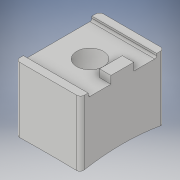
# Autodesk Inventor part: upper_fender_spacer
Saved by Autodesk Inventor 2019 (Build 230136000, 136)
## iProperties
Created: 2019-10-03
Part Number: upper_fender_spacer
Material: Generic
Document SubType Name: Modeling
Designer: Alex
Density: 1 g/cm^3
Appearance: Default
Author: Alex
Autodesk Inventor part; units mm, degrees
ref_plane "YZ Plane" through (0, 0, 0) normal (1, 0, 0) x (0, 1, 0)
ref_plane "XZ Plane" through (0, 0, 0) normal (0, 1, 0) x (-1, 0, 0)
ref_plane "XY Plane" through (0, 0, 0) normal (0, 0, 1) x (1, 0, 0)
sketch "Sketch1" plane through (0, 0, 0) normal (0, 1, 0) x (-1, 0, 0)
  line L0 (5.233, 7.4455) -> (-11.767, 7.4455)
  line L1 (-11.767, 7.4455) -> (-11.767, -14.5545)
  line L2 (-11.767, -14.5545) -> (5.233, -14.5545)
  circle A0 centre (-3.267, -3.5545) radius 3.5
  line L3 (5.233, 7.4455) -> (5.233, -14.5545)
  point P0 (0, 0)
  dimension "d2" = 22
  dimension "d3" = 17
  dimension "d8" = 7
  dimension "d10" = 11
  dimension "d11" = 8.5
  constraints: 8 end point, 1 centre point, 1 horizontal, 1 parallel, 1 perpendicular, 1 vertical
  measures "d2" distance of L2.end L0.start
  measures "d3" distance of L0.start L0.end
  measures "d8" diameter of A0
  measures "d10" distance from line of A0.centre L0
  measures "d11" distance from line of A0.centre L3
extrude "Extrusion1" add sketch "Sketch1" along normal blind 20
sketch "Sketch2" plane through (0, 20, 0) normal (0, 1, 0) x (1, 0, 0)
  line L0 (-5.233, -7.4455) -> (11.767, -7.4455) projected
  line L1 (11.767, -7.4455) -> (11.767, 14.5545) projected
  line L2 (-5.233, -7.4455) -> (11.767, -7.4455)
  line L3 (11.767, -7.4455) -> (11.767, -5.4455)
  line L4 (11.767, -5.4455) -> (-5.233, -5.4455)
  line L5 (-5.233, -5.4455) -> (-5.233, -7.4455)
  line L6 (-5.233, 14.5545) -> (-5.233, -7.4455) projected
  line L7 (-5.233, 14.5545) -> (11.767, 14.5545)
  line L8 (11.767, 14.5545) -> (11.767, 12.5545)
  line L9 (11.767, 12.5545) -> (-5.233, 12.5545)
  line L10 (-5.233, 12.5545) -> (-5.233, 14.5545)
  line L11 (11.767, 0.5545) -> (8.767, 0.5545)
  line L12 (8.767, 0.5545) -> (8.767, 6.5545)
  line L13 (8.767, 6.5545) -> (11.767, 6.5545)
  line L14 (11.767, 6.5545) -> (11.767, 0.5545)
  line L15 (11.767, 0.5545) -> (8.767, 0.5545)
  line L16 (8.767, 0.5545) -> (8.767, 6.5545)
  line L17 (8.767, 6.5545) -> (11.767, 6.5545)
  line L18 (11.767, 6.5545) -> (11.767, 0.5545)
  point P0 (0, 0)
  dimension "d14" = 2
  dimension "d15" = 2
  dimension "d16" = 3
  dimension "d17" = 6
  dimension "d18" = 8
  constraints: 32 end point, 8 parallel, 4 horizontal, 4 perpendicular, 3 point on line
  measures "d14" distance between parallel lines of L4 L0
  measures "d15" distance between parallel lines of L7 L9
  measures "d16" distance between parallel lines of L1 L12
  measures "d17" distance between parallel lines of L11 L13
  measures "d18" distance between parallel lines of L11 L0
extrude "Extrusion2" add sketch "Sketch2" along normal blind 1 contours L5 L4 L1 L0 | L6 L7 L1 L9
sketch "Sketch3" plane through (0, 20, 0) normal (0, 1, 0) x (1, 0, 0)
  line L0 (11.767, -5.4455) -> (11.767, 12.5545) projected
  line L1 (11.767, 0.5545) -> (8.767, 0.5545)
  line L2 (8.767, 0.5545) -> (8.767, 6.5545)
  line L3 (8.767, 6.5545) -> (11.767, 6.5545)
  line L4 (11.767, 6.5545) -> (11.767, 0.5545)
  line L5 (-5.233, -7.4455) -> (11.767, -7.4455) projected
  point P0 (0, 0)
  dimension "d21" = 6
  dimension "d22" = 3
  dimension "d23" = 8
  constraints: 8 end point, 2 parallel, 1 horizontal, 1 perpendicular, 1 point on line
  measures "d21" distance between parallel lines of L3 L1
  measures "d22" distance between parallel lines of L0 L2
  measures "d23" distance between parallel lines of L1 L5
extrude "Extrusion3" add sketch "Sketch3" along normal blind 2
sketch "Sketch5" plane through (-5.233, 0, -14.5545) normal (-1, 0, 0) x (0, 0, 1)
  line L0 (-21.5, -5) -> (43.5, -5)
  line L1 (11, -5) -> (11, 5)
  line L2 (0, 0) -> (0, 21) projected
  arc A0 (43.5, -5) -> (22, 3.9439) centre (11, -52.8125) ccw
  line L3 (2, 20) -> (20, 20) projected
  arc A1 (11, 5) -> (-21.5, -5) centre (11, -52.8125) ccw
  arc A2 (0, 3.9439) -> (-21.5, -5) centre (11, -52.8125) ccw
  line L4 (0, 0) -> (22, 0) projected
  line L5 (22, 0) -> (22, 3.9439)
  line L6 (22, 0) -> (0, 0)
  line L7 (0, 0) -> (0, 3.9439)
  arc A3 (22, 3.9439) -> (11, 5) centre (11, -52.8125) ccw
  line L8 (-15.7774, -378) -> (53.3664, -378)
  point P0 (14.5545, 0)
  dimension "d27" = 65
  dimension "d28" = 10
  dimension "d29" = 32.5
  dimension "d30" = 21.5
  dimension "d31" = 15
  dimension "d32" = 373
  constraints: 10 end point, 9 point on circle, 4 centre point, 2 perpendicular, 1 collinear, 1 horizontal, 1 point on line, 1 vertical, 4 other
  measures "d27" distance of A1.end A0.start
  measures "d28" distance of L1.start L1.end
  measures "d29" distance from line of A1.end L1
  measures "d30" distance from line of A1.end L2
  measures "d31" distance from line of L3 L1.end
move or copy body "Move Body1" bodies to move or copy 1 copy no translate (-8.5, 0, 0)
revolve "Revolution1" cut sketch "Sketch5" angle 360 about axis through (-5.233, -378, -30.3319) along (0, 0, 1)
fillet "Fillet1" radius 1 4 edges at (-13.733, 12.4246, -14.5545) (3.267, 12.4246, -14.5545) (-13.733, 12.4246, 7.4455) (3.267, 12.4246, 7.4455)
fillet "Fillet2" radius 0.5 1 edges at (-5.233, 20, -12.5545)
fillet "Fillet3" radius 0.5 1 edges at (-5.233, 20, 5.4455)
body "Solid1"
